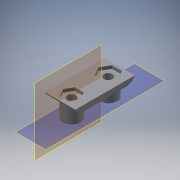
# Autodesk Inventor part: Isolationsmasse
Saved by Autodesk Inventor 2017 (Build 210142000, 142)
## iProperties
Part Number: Isolationsmasse
Material: Generisch
Document SubType Name: Modeling
Designer: David Merges
Density: 1 g/cm^3
Appearance: Vorgabe
Author: David Merges
Autodesk Inventor part; units mm, degrees
ref_plane "XZ Plane" through (0, 0, 0) normal (0, 1, 0) x (-1, 0, 0)
ref_plane "XY Plane" through (0, 0, 0) normal (0, 0, 1) x (1, 0, 0)
ref_plane "Arbeitsebene1" through (5, 7.0959, 0) normal (1, 0, 0) x (0, 1, 0)
sketch "Skizze1" plane through (5, 7.0959, 0) normal (1, 0, 0) x (0, 1, 0)
  arc A0 (6.9041, 0) -> (9.9041, 3) centre (6.9041, 3) ccw projected
  line L0 (6.9041, 0) -> (-7.0959, 0) projected
  arc A1 (-10.0959, 3) -> (-7.0959, 0) centre (-7.0959, 3) ccw projected
  line L1 (9.6536, 1.8) -> (-9.8455, 1.8)
  dimension "d0" = 1.8
  constraints: 2 end point, 2 point on circle, 1 horizontal
  measures "d0" distance between parallel lines of L1 L0
extrude "Extrusion1" add sketch "Skizze1" along normal mid plane 10
ref_plane "Arbeitsebene2" through (5, -12.9041, -4.7) normal (0, 0, -1) x (-1, 0, 0)
sketch "Skizze2" plane through (5, -12.9041, -4.7) normal (0, 0, -1) x (-1, 0, 0)
  arc A0 (-2.8982, 26.7749) -> (2.8982, 26.7749) centre (0, 26) ccw projected
  arc A1 (2.7927, 12.9041) -> (-2.7927, 12.9041) centre (0, 14) ccw projected
  circle A2 centre (0, 14) radius 3
  circle A3 centre (0, 26) radius 3
  circle A4 centre (0, 26) radius 2
  circle A5 centre (0, 14) radius 2
  point P0 (5, 12.9041)
  dimension "d3" = 0
  dimension "d4" = 4
  constraints: 4 centre point, 4 coincident, 2 equal radius
  measures "d3" radial gap between concentric circles of A1 A2
  measures "d4" diameter of A5
extrude "Extrusion2" add sketch "Skizze2" against normal up to surface (6.5 mm away)
sketch "Skizze3" plane through (5, 13.0959, -4.7) normal (0, 0, -1) x (-1, 0, 0)
  circle A0 centre (0, 0) radius 2 projected
  circle A1 centre (0, -12) radius 2 projected
  point P0 (5, -13.0959)
extrude "Extrusion3" cut sketch "Skizze3" against normal up to surface (6.5 mm away)
sketch "Skizze4" plane through (0, -2.7495, 1.8) normal (0, 0, 1) x (1, 0, 0)
  circle A0 centre (5, 15.8455) radius 2 projected
  circle A1 centre (5, 3.8455) radius 2 projected
  line L0 (0, 0) -> (10, 0) projected
  line L1 (10, 19.4991) -> (10, 0) projected
  line L2 (0, 19.4991) -> (10, 19.4991) projected
  line L3 (0, 0) -> (0, 19.4991) projected
  circle A2 centre (5, 15.8455) radius 2 projected
  line L4 (7.8866, 15.8762) -> (6.4699, 13.361)
  line L5 (6.4699, 13.361) -> (3.5833, 13.3303)
  line L6 (3.5833, 13.3303) -> (2.1134, 15.8148)
  line L7 (2.1134, 15.8148) -> (3.5301, 18.33)
  line L8 (3.5301, 18.33) -> (6.4167, 18.3607)
  line L9 (6.4167, 18.3607) -> (7.8866, 15.8762)
  line L10 (7.8866, 3.8762) -> (6.4699, 1.361)
  line L11 (6.4699, 1.361) -> (3.5833, 1.3303)
  line L12 (3.5833, 1.3303) -> (2.1134, 3.8148)
  line L13 (2.1134, 3.8148) -> (3.5301, 6.33)
  line L14 (3.5301, 6.33) -> (6.4167, 6.3607)
  line L15 (6.4167, 6.3607) -> (7.8866, 3.8762)
  point P0 (0, 2.7495)
  dimension "d9" = 5
  constraints: 24 end point, 2 coincident, 2 parallel, 26 other
  measures "d9" distance between parallel lines of L10 L13
extrude "Extrusion4" cut sketch "Skizze4" against normal blind 1 contours L4 L5 L6 L7 L8 L9 | L10 L11 L12 L13 L14 L15
